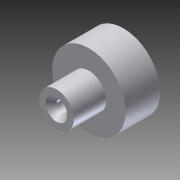
# Autodesk Inventor part: MU_Bearing_Housing2
Saved by Autodesk Inventor 2011 SP2 (Build 150309200, 309)
## iProperties
Created: 2011-01-18
Part Number: MU_Bearing_Housing2
Document SubType Name: Modeling
Designer: sungwook
Density: 2.71 g/cm^3
Material: Aluminum-6061-AHC
Mass: 0.0275156 g
Surface Area: 0.550491 cm^2
Volume: 0.0101534 cm^3
Author: sungwook
Autodesk Inventor part; units mm, degrees
ref_plane "YZ Plane" through (0, 0, 0) normal (1, 0, 0) x (0, 1, 0)
ref_plane "XZ Plane" through (0, 0, 0) normal (0, 1, 0) x (-1, 0, 0)
ref_plane "XY Plane" through (0, 0, 0) normal (0, 0, 1) x (1, 0, 0)
sketch "Sketch1" plane through (0, 0, 0) normal (0, 0, 1) x (1, 0, 0)
  circle A0 centre (0, 0) radius 1.7
  dimension "d0" = 3.4
  constraints: 1 centre point, 1 coincident
  measures "d0" diameter of A0
extrude "Extrusion1" add sketch "Sketch1" along normal blind 3.1
sketch "Sketch2" plane through (0, 0, 3.1) normal (0, 0, 1) x (1, 0, 0)
  circle A0 centre (0, 0) radius 1.7 projected
  circle A1 centre (0, 0) radius 0.2
  dimension "d3" = 0.4
  constraints: 1 centre point, 1 coincident
  measures "d3" diameter of A1
extrude "Extrusion2" [suppressed]
sketch "Sketch3" plane through (0, 0, 0) normal (0, 0, -1) x (-1, 0, 0)
  circle A0 centre (0, 0) radius 1.7 projected
  circle A1 centre (0, 0) radius 1.5
  dimension "d6" = 3
  constraints: 1 centre point, 1 coincident
  measures "d6" diameter of A1
extrude "Extrusion3" cut sketch "Sketch3" against normal blind 0.9 contours A1
sketch "Sketch4" plane through (0, 0, 3.1) normal (0, 0, 1) x (1, 0, 0)
  circle A0 centre (0, 0) radius 1.7 projected
  circle A1 centre (0, 0) radius 0.8
  dimension "d9" = 1.6
  constraints: 1 centre point, 1 coincident
  measures "d9" diameter of A1
extrude "Extrusion4" cut sketch "Sketch4" against normal blind 1.5
sketch "Sketch5" plane through (0, 0, 0.9) normal (0, 0, -1) x (-1, 0, 0)
  circle A0 centre (0, 0) radius 1.5 projected
  circle A1 centre (0, 0) radius 1.5 projected
  circle A2 centre (0, 0) radius 1.5 projected
  circle A3 centre (0, 0) radius 0.65
  dimension "d12" = 3
  dimension "d13" = 1.3
  constraints: 1 centre point, 1 coincident
  measures "d12" diameter of A0
  measures "d13" diameter of A3
extrude "Extrusion5" [suppressed]
chamfer "Chamfer1" [suppressed]
hole "Hole1" at (0, 0, 3.1) direction (0, 0, -1) diameter 0.5 depth 1.7 countersink diameter 1 countersink angle 90
sketch "Sketch6" plane through (0, 0, 0.9) normal (0, 0, -1) x (-1, 0, 0)
  circle A0 centre (0, 0) radius 1.5 projected
  circle A1 centre (0, 0) radius 1.5 projected
  circle A2 centre (0, 0) radius 1
  dimension "d28" = 2
  constraints: 1 centre point, 1 coincident
  measures "d28" diameter of A2
extrude "Extrusion6" cut sketch "Sketch6" against normal blind 0.2 contours A2
equation "\"baseInitD\" = 4"
equation "\"baseTh0\" = 48.463041deg"
equation "\"baseTh1\" = 23.073918deg"
equation "\"topD\" = 14"
equation "\"topInitD\" = 4"
equation "\"topTh0\" = 16.60155deg"
equation "\"topTh1\" = 86.796901deg"
equation "\"dFlexure\" = 0.38"
equation "\"lFlexure\" = 1.5"
equation "\"springBaseD\" = 8"
equation "\"dMotor\" = 1.44"
equation "\"springTopD\" = 8"
equation "\"springInitL\" = 12.7"
equation "\"lMotor\" = 22.35"
equation "\"topH\" = 21.66629"
equation "\"springL\" = 30.86629"
equation "\"springLset\" = 3.5"
equation "\"springDeform\" = 18.16629"
equation "\"springUnderCut\" = 9.2"
equation "\"spirngLO\" = 31.67176"
equation "\"springLO\" = 33.86629"
equation "\"lFlexureOffset\" = 1.95"
equation "\"dM2X\" = -1.34133"
equation "\"dM2Y\" = 7.00349"
equation "\"dM1Y\" = 2.34012"
equation "\"dM1X\" = 6.73587"
equation "\"dM1Yt\" = -0.43704"
equation "\"dM1Xt\" = 6.59227"
equation "\"dM2Xt\" = -3.67462"
equation "\"dM2Yt\" = 5.49055"
equation "\"GuideRod\" = 2"
equation "\"baseOD\" = 23"
equation "\"CSpringOD\" = 5.537"
equation "\"GuideTubingOD\" = 4"
equation "\"CSpringID\" = 5.029"
equation "\"CSpringCD\" = 0.254"
equation "\"GuideTubingID\" = 2"
equation "\"lOCTprobe\" = 1905"
equation "\"OCToffset\" = 365.252"
equation "\"lOCT\" = 1473.2"
equation "\"lOCTprobeNorm\" = 1838.452"
equation "\"lOCTprobeNom\" = 1838.452"
equation "\"OCTd0\" = 508"
equation "\"OCTd1\" = 254"
body "Solid1"
